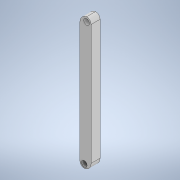
# Autodesk Inventor part: rod
Saved by Autodesk Inventor 2021 (Build 250183000, 183)
## iProperties
Created: 2021-02-01
Part Number: rod
Material: Generic
Document SubType Name: Modeling
Designer: chris
Density: 1 g/cm^3
Appearance: Default
Author: chris
Autodesk Inventor part; units mm, degrees
ref_plane "YZ Plane" through (0, 0, 0) normal (1, 0, 0) x (0, 1, 0)
ref_plane "XZ Plane" through (0, 0, 0) normal (0, 1, 0) x (-1, 0, 0)
ref_plane "XY Plane" through (0, 0, 0) normal (0, 0, 1) x (1, 0, 0)
sketch "Sketch1" plane through (0, 0, 0) normal (0, 0, 1) x (1, 0, 0)
  line L0 (0, 0) -> (10, 0)
  line L1 (10, 0) -> (10, 118.5)
  line L2 (10, 118.5) -> (0, 118.5)
  line L3 (0, 118.5) -> (0, 0)
  dimension "d1" = 10
  dimension "d14" = 118.5
  constraints: 8 end point, 2 parallel, 1 horizontal, 1 perpendicular
  measures "d1" distance of L1.end L2.end
  measures "d14" distance between parallel lines of L0 L2
extrude "Extrusion1" add sketch "Sketch1" along normal blind 8
sketch "Sketch2" plane through (0, 0, 8) normal (0, 0, 1) x (1, 0, 0)
  circle A0 centre (3.9473, 3.5528) radius 2.5
  circle A1 centre (6.4473, 196.4185) radius 2.5
  point P0 (0, 0)
  dimension "d4" = 5
  dimension "d5" = 5
  constraints: 2 centre point
  measures "d4" diameter of A0
  measures "d5" diameter of A1
extrude "Extrusion2" cut sketch "Sketch2" against normal through all
sketch "Sketch3" plane through (0, 0, 8) normal (0, 0, 1) x (1, 0, 0)
  circle A0 centre (6, 114.5) radius 2.5
  line L0 (10, 118.5) -> (0, 118.5) projected
  line L1 (10, 0) -> (10, 118.5) projected
  point P0 (0, 0)
  dimension "d8" = 5
  dimension "d9" = 4
  dimension "d10" = 4
  constraints: 1 centre point
  measures "d8" diameter of A0
  measures "d9" distance from line of L0 A0.centre
  measures "d10" distance from line of L1 A0.centre
extrude "Extrusion3" cut sketch "Sketch3" against normal through all
fillet "Fillet3" radius 4 2 edges at (10, 118.5, 4) (0, 0, 4)
fillet "Fillet4" radius 7 2 edges at (10, 0, 4) (0, 118.5, 4)
body "Solid1"
